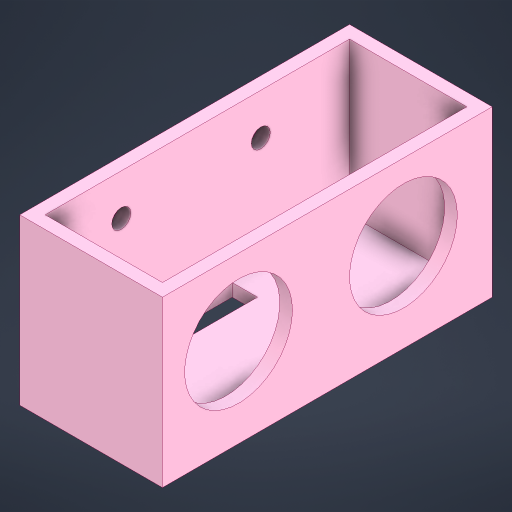
# Autodesk Inventor part: soporte_sensor
Saved by Autodesk Inventor 2023.1 (Build 271208000, 208)
## iProperties
Created: 2022-10-26
Part Number: soporte_sensor
Material: Generic
Document SubType Name: Modeling
Designer: amtat
Density: 1 g/cm^3
Appearance: Default
Author: amtat
Autodesk Inventor part; units mm, degrees
ref_plane "YZ Plane" through (0, 0, 0) normal (1, 0, 0) x (0, 1, 0)
ref_plane "XZ Plane" through (0, 0, 0) normal (0, 1, 0) x (-1, 0, 0)
ref_plane "XY Plane" through (0, 0, 0) normal (0, 0, 1) x (1, 0, 0)
sketch "Sketch1" plane through (0, 0, 0) normal (1, 0, 0) x (0, 1, 0)
  line L0 (0, 0) -> (0, -52)
  line L1 (0, -52) -> (26, -52)
  line L2 (26, -52) -> (26, 0)
  line L3 (26, 0) -> (0, 0)
  line L4 (26, 0) -> (19.5, 0)
  line L5 (19.5, 0) -> (19.5, -14)
  line L6 (19.5, -14) -> (19.5, -36)
  circle A0 centre (19.5, -14) radius 1.5
  circle A1 centre (19.5, -36) radius 1.5
  dimension "d0" = 52
  dimension "d1" = 26
  dimension "d2" = 6.5
  dimension "d3" = 14
  dimension "d4" = 22
  dimension "d5" = 3
  dimension "d6" = 3
  constraints: 14 end point, 3 perpendicular, 2 centre point, 2 coincident, 2 vertical, 1 horizontal, 1 point on line
  measures "d0" distance of L0.start L0.end
  measures "d1" distance of L0.end L1.end
  measures "d2" distance of L2.end L4.end
  measures "d3" distance of L4.end L5.end
  measures "d4" distance of L5.end L6.end
  measures "d5" diameter of A0
  measures "d6" diameter of A1
extrude "Extrusion1" add sketch "Sketch1" along normal blind 2
sketch "Sketch2" plane through (2, 0, 0) normal (1, 0, 0) x (0, 0, -1)
  line L0 (0, 0) -> (52, 0) projected
  line L1 (52, 0) -> (52, 26) projected
  line L2 (52, 26) -> (0, 26) projected
  line L3 (0, 26) -> (0, 0) projected
  circle A0 centre (36, 19.5) radius 1.5 projected
  circle A1 centre (14, 19.5) radius 1.5 projected
  line L4 (52, 26) -> (0, 26) projected
  line L5 (0, 26) -> (2, 26)
  line L6 (2, 26) -> (2, 2)
  line L7 (2, 2) -> (50, 2)
  line L8 (50, 2) -> (50, 24)
  line L9 (50, 24) -> (2, 24)
  line L10 (50, 24) -> (50, 26)
  dimension "d9" = 2
  dimension "d10" = 24
  dimension "d11" = 48
  dimension "d12" = 22
  constraints: 12 end point, 5 perpendicular, 3 point on line
  measures "d9" distance of L2.end L5.end
  measures "d10" distance of L5.end L6.end
  measures "d11" distance of L6.end L7.end
  measures "d12" distance of L7.end L8.end
extrude "Extrusion2" add sketch "Sketch2" along normal blind 17 contours L3 L2 L6 L7 L8 L10 L1 L0
sketch "Sketch3" plane through (19, 0, 0) normal (1, 0, 0) x (0, 0, -1)
  line L0 (52, 26) -> (50, 26) projected
  line L1 (50, 26) -> (50, 2) projected
  line L2 (50, 2) -> (2, 2) projected
  line L3 (2, 2) -> (2, 26) projected
  line L4 (2, 26) -> (0, 26) projected
  line L5 (0, 26) -> (0, 0) projected
  line L6 (0, 0) -> (52, 0) projected
  line L7 (52, 0) -> (52, 26) projected
  line L8 (2, 26) -> (0, 26) projected
  line L9 (52, 26) -> (0, 26) projected
  line L10 (0, 26) -> (52, 26)
  constraints: 2 end point, 1 collinear
extrude "Extrusion3" add sketch "Sketch3" along normal blind 2
sketch "Sketch4" plane through (21, 0, 0) normal (1, 0, 0) x (0, 0, -1)
  circle A0 centre (14, 19.5) radius 1.5 projected
  line L0 (52, 26) -> (0, 26) projected
  line L1 (0, 26) -> (0, 0) projected
  line L2 (0, 0) -> (52, 0) projected
  line L3 (52, 0) -> (52, 26) projected
  circle A1 centre (36, 19.5) radius 1.5 projected
  line L4 (52, 26) -> (0, 26) projected
  line L5 (0, 26) -> (0, 0) projected
  line L6 (0, 0) -> (52, 0) projected
  line L7 (52, 0) -> (52, 26) projected
  line L8 (0, 26) -> (0, 0) projected
  line L9 (0, 26) -> (25, 26)
  line L10 (50, 26) -> (2, 26) projected
  line L11 (25, 26) -> (38, 26)
  line L12 (38, 26) -> (38, 0)
  line L13 (0, 0) -> (52, 0) projected
  line L14 (25, 26) -> (12, 26)
  line L15 (12, 26) -> (12, 0)
  line L16 (52, 26) -> (0, 26) projected
  line L17 (0, 26) -> (0, 4)
  line L18 (0, 4) -> (50, 4)
  line L19 (52, 0) -> (52, 26) projected
  line L20 (50, 4) -> (50, 26)
  line L21 (0, 26) -> (0, 24)
  line L22 (0, 24) -> (0, 14)
  line L23 (0, 14) -> (38, 14)
  circle A2 centre (12, 14) radius 8.5
  circle A3 centre (38, 14) radius 8.5
  dimension "d17" = 25
  dimension "d18" = 13
  dimension "d19" = 13
  dimension "d20" = 22
  dimension "d21" = 2
  dimension "d22" = 10
  dimension "d23" = 17
  dimension "d24" = 17
  constraints: 22 end point, 11 point on line, 5 perpendicular, 2 centre point, 1 coincident, 1 other
  measures "d17" distance of L0.end L9.end
  measures "d18" distance of L9.end L11.end
  measures "d19" distance of L9.end L14.end
  measures "d20" distance of L0.end L17.end
  measures "d21" distance of L4.end L21.end
  measures "d22" distance of L21.end L22.end
  measures "d23" diameter of A2
  measures "d24" diameter of A3
extrude "Extrusion4" cut sketch "Sketch4" against normal blind 2 contours A0 | A3 L12 | L12 L23 A3 | L12 A3 L23 | A2 L23 L15 | L15 L23 A2 | A2 L15 L23 | A2 L23 L15 | A1
sketch "Sketch5" plane through (2, 2, -2) normal (0, 1, 0) x (1, 0, 0)
  line L0 (0, 0) -> (0, 48) projected
  line L1 (0, 0) -> (17, 0) projected
  line L2 (17, 48) -> (17, 0) projected
  line L3 (0, 48) -> (17, 48) projected
  line L4 (0, 13.5) -> (0, 10.5) projected
  line L5 (0, 35.5) -> (0, 32.5) projected
  line L6 (0, 48) -> (0, 0) projected
  line L7 (0, 0) -> (0, 12)
  line L8 (0, 12) -> (0, 34)
  line L9 (0, 12) -> (0, 23)
  line L10 (0, 23) -> (0, 29.5)
  line L11 (0, 29.5) -> (4, 29.5)
  line L12 (4, 29.5) -> (4, 16.5)
  line L13 (4, 16.5) -> (0, 16.5)
  line L14 (0, 16.5) -> (0, 23)
  point P0 (-2, -2)
  point P1 (0, 16.5)
  dimension "d27" = 12
  dimension "d28" = 22
  dimension "d29" = 11
  dimension "d30" = 6.5
  dimension "d31" = 4
  dimension "d32" = 13
  constraints: 16 end point, 4 point on line, 3 perpendicular, 1 collinear, 1 midpoint
  measures "d27" distance of L0.start L7.end
  measures "d28" distance of L7.end L8.end
  measures "d29" distance of L7.end L9.end
  measures "d30" distance of L9.end L10.end
  measures "d31" distance of L10.end L11.end
  measures "d32" distance of L11.end L12.end
extrude "Extrusion5" cut sketch "Sketch5" against normal blind 2 contours L0 L11 L12 L13
sketch "Sketch6" plane through (21, 0, 0) normal (1, 0, 0) x (0, 0, -1)
  circle A0 centre (38, 14) radius 8.5 projected
  circle A1 centre (12, 14) radius 8.5 projected
  line L0 (52, 26) -> (0, 26) projected
  line L1 (0, 26) -> (0, 0) projected
  line L2 (0, 0) -> (52, 0) projected
  line L3 (52, 0) -> (52, 26) projected
extrude "Extrusion6" add sketch "Sketch6" along normal blind 1.5
sketch "Sketch7" plane through (19, 0, 0) normal (-1, 0, 0) x (0, 0, 1)
  line L0 (0, 26) -> (0, 0) projected
  line L1 (0, 0) -> (-52, 0) projected
  line L2 (-52, 0) -> (-52, 26) projected
  line L3 (-52, 26) -> (0, 26) projected
  circle A0 centre (-38, 14) radius 8.5 projected
  circle A1 centre (-12, 14) radius 8.5 projected
  line L4 (0, 26) -> (0, 0) projected
  line L5 (0, 26) -> (-2, 26)
  line L6 (-52, 26) -> (0, 26) projected
  line L7 (-2, 26) -> (-2, 2)
  line L8 (-2, 2) -> (-50, 2)
  line L9 (-50, 2) -> (-50, 26)
  dimension "d37" = 2
  dimension "d38" = 24
  dimension "d39" = 48
  constraints: 8 end point, 3 perpendicular, 2 point on line
  measures "d37" distance of L0.start L5.end
  measures "d38" distance of L5.end L7.end
  measures "d39" distance of L7.end L8.end
extrude "Extrusion7" cut sketch "Sketch7" against normal blind 1.5 contours L7 L8 L9 L3
body "Solid1"
